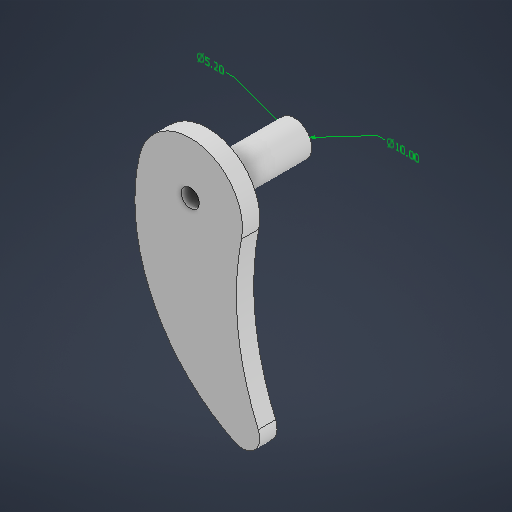
# Autodesk Inventor part: p2
Saved by Autodesk Inventor 2026.2 (Build 302298010, 298A)
## iProperties
Created: 2026-03-23
Part Number: p2
Material: Generic
Document SubType Name: Modeling
Designer: anasa
Density: 1 g/cm^3
Appearance: Default
Author: anasa
## iProperties of the stored document p2_3DPrint.ipt
Created: 2026-04-19
Part Number: p2_3DPrint
Material: Generic
Document SubType Name: Modeling
Designer: lenovo
Density: 1 g/cm^3
Appearance: Default
Author: lenovo
Autodesk Inventor part; units mm, degrees
ref_plane "YZ Plane" through (0, 0, 0) normal (1, 0, 0) x (0, 1, 0)
ref_plane "XZ Plane" through (0, 0, 0) normal (0, 1, 0) x (-1, 0, 0)
ref_plane "XY Plane" through (0, 0, 0) normal (0, 0, 1) x (1, 0, 0)
sketch "Sketch1" plane through (0, 0, 0) normal (0, 0, 1) x (1, 0, 0)
  circle A0 centre (0, 0) radius 15
  circle A1 centre (15, -50) radius 5
  arc A2 (14.7146, -2.9124) -> (19.5845, -48.0044) centre (89.2722, -17.6691) ccw
  arc A3 (-14.5962, 3.4571) -> (12.8032, -54.4915) centre (35.3589, -8.3749) ccw
  point P0 (15, -55)
  point P1 (13.6233, -6.2774)
  point P2 (15, -45)
  dimension "d0" = 30
  dimension "d1" = 10
  dimension "d2" = 15
  dimension "d3" = 50
  constraints: 11 point on circle, 4 centre point, 4 tangent, 1 coincident
  measures "d0" diameter of A0
  measures "d1" diameter of A1
  measures "d2" horizontal distance of A1.centre point (0, 0)
  measures "d3" vertical distance of point (0, 0) A1.centre
extrude "Extrusion1" add sketch "Sketch1" along normal blind 5
sketch "Sketch2" plane through (0, 0, 5) normal (0, 0, 1) x (1, 0, 0)
  circle A0 centre (0, 0) radius 2.6
  dimension "d8" = 5.2
  constraints: 1 centre point, 1 coincident
  measures "d8" diameter of A0
extrude "Extrusion2" cut sketch "Sketch2" against normal blind 40
sketch "Sketch3" plane through (0, 0, 0) normal (0, 0, -1) x (-1, 0, 0)
  circle A0 centre (0, 0) radius 2.6 projected
  circle A1 centre (0, 0) radius 5
  circle A2 centre (0, 0) radius 2.6
  dimension "d13" = 10
  constraints: 2 centre point, 2 coincident, 1 concentric
  measures "d13" diameter of A1
extrude "Extrusion3" add sketch "Sketch3" along normal blind 25
body "Solid1"
